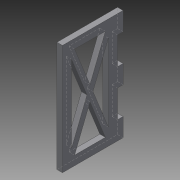
# Autodesk Inventor part: Back Plate
Saved by Autodesk Inventor 2015 (Build 190159000, 159)
## iProperties
Created: 2014-07-28
Part Number: Back Plate
Material: Generic
Document SubType Name: Modeling
Designer: karl
Density: 1 g/cm^3
Appearance: Default
Author: karl
Autodesk Inventor part; units mm, degrees
ref_plane "YZ Plane" through (0, 0, 0) normal (1, 0, 0) x (0, 1, 0)
ref_plane "XZ Plane" through (0, 0, 0) normal (0, 1, 0) x (-1, 0, 0)
ref_plane "XY Plane" through (0, 0, 0) normal (0, 0, 1) x (1, 0, 0)
sketch "Sketch1" plane through (0, 0, 0) normal (1, 0, 0) x (0, 1, 0)
  line L0 (15, 30) -> (-15, 30)
  line L1 (-15, 30) -> (-15, -30)
  line L2 (-15, -30) -> (15, -30)
  line L3 (15, -30) -> (15, 30)
  line L4 (15, 30) -> (-15, -30) construction
  line L5 (-15, 30) -> (15, -30) construction
  line L6 (15, 30) -> (18, 30)
  line L7 (18, 30) -> (18, 20)
  line L8 (18, 20) -> (15, 20)
  line L9 (15, 20) -> (15, 30)
  line L10 (15, -30) -> (18, -30)
  line L11 (18, -30) -> (18, -20)
  line L12 (18, -20) -> (15, -20)
  line L13 (15, -20) -> (15, -30)
  line L14 (15, 5) -> (18, 5)
  line L15 (18, 5) -> (18, -5)
  line L16 (18, -5) -> (15, -5)
  line L17 (15, -5) -> (15, 5)
  point P0 (0, 0)
  point P1 (18, 0)
  point P2 (0, 0)
  dimension "d0" = 30
  dimension "d1" = 60
  dimension "d2" = 3
  dimension "d3" = 10
  dimension "d4" = 3
  dimension "d5" = 10
  dimension "d6" = 3
  dimension "d7" = 10
  constraints: 36 end point, 8 parallel, 4 horizontal, 4 midpoint, 4 perpendicular, 1 horizontal alignment, 1 point on line
  measures "d0" distance of L2.end L1.end
  measures "d1" distance of L0.end L1.end
  measures "d2" distance of L7.end L8.end
  measures "d3" distance of L6.end L7.end
  measures "d4" distance of L12.end L11.end
  measures "d5" distance of L11.end L10.end
  measures "d6" distance of L15.end L16.end
  measures "d7" distance of L14.end L15.end
extrude "Extrusion1" add sketch "Sketch1" along normal blind 3
sketch "Sketch2" plane through (0, 0, 0) normal (-1, 0, 0) x (0, 0, 1)
  line L0 (25, 10) -> (-25, 10)
  line L1 (-25, 10) -> (-25, -10)
  line L2 (-25, -10) -> (25, -10)
  line L3 (25, -10) -> (25, 10)
  line L4 (25, 10) -> (-25, -10) construction
  line L5 (-25, 10) -> (25, -10) construction
  line L6 (30, -15) -> (-30, -15) projected
  line L7 (-30, -15) -> (-30, 18) projected
  point P0 (0, 0)
  dimension "d10" = 5
  dimension "d11" = 5
  constraints: 12 end point, 2 midpoint, 2 parallel, 1 horizontal, 1 perpendicular
  measures "d10" distance between parallel lines of L6 L2
  measures "d11" distance between parallel lines of L7 L1
extrude "Extrusion2" cut sketch "Sketch2" against normal blind 3
sketch "Sketch3" plane through (0, 0, 0) normal (-1, 0, 0) x (0, 0, 1)
  line L0 (-25, -10) -> (-25, 10) projected
  line L1 (-25, 10) -> (25, 10) projected
  line L2 (25, 10) -> (25, -10) projected
  line L3 (25, -10) -> (-25, -10) projected
  line L4 (-30, -15) -> (-30, 18) projected
  line L5 (30, -15) -> (-30, -15) projected
  line L6 (30, 18) -> (30, -15) projected
  line L7 (20, 18) -> (30, 18) projected
  line L8 (20, 15) -> (20, 18) projected
  line L9 (5, 15) -> (20, 15) projected
  line L10 (5, 18) -> (5, 15) projected
  line L11 (-5, 18) -> (5, 18) projected
  line L12 (-5, 15) -> (-5, 18) projected
  line L13 (-20, 15) -> (-5, 15) projected
  line L14 (-20, 18) -> (-20, 15) projected
  line L15 (-30, 18) -> (-20, 18) projected
  line L16 (25.5571, 8.6073) -> (-24.4429, -11.3927)
  line L17 (-24.4429, -11.3927) -> (-25.5571, -8.6073)
  line L18 (-25.5571, -8.6073) -> (24.4429, 11.3927)
  line L19 (24.4429, 11.3927) -> (25.5571, 8.6073)
  line L20 (25.5571, 8.6073) -> (-25.5571, -8.6073) construction
  line L21 (-24.4429, -11.3927) -> (24.4429, 11.3927) construction
  line L22 (-25.5571, 8.6073) -> (24.4429, -11.3927)
  line L23 (24.4429, -11.3927) -> (25.5571, -8.6073)
  line L24 (25.5571, -8.6073) -> (-24.4429, 11.3927)
  line L25 (-24.4429, 11.3927) -> (-25.5571, 8.6073)
  line L26 (-25.5571, 8.6073) -> (25.5571, -8.6073) construction
  line L27 (24.4429, -11.3927) -> (-24.4429, 11.3927) construction
  point P0 (0, 0)
  dimension "d14" = 3
  dimension "d15" = 3
  constraints: 24 end point, 4 midpoint, 4 parallel, 2 perpendicular
  measures "d14" distance of L16.end L17.end
  measures "d15" distance of L23.end L22.end
extrude "Extrusion3" add sketch "Sketch3" against normal blind 3 contours L17 L18 L0 | L0 L18 L22 L16 L3 | L3 L16 L17 | L22 L25 L0 | L0 L1 L24 L18 L22 | L18 L24 L16 L22 | L22 L16 L24 L2 L3 | L3 L23 L22 | L25 L24 L1 | L18 L1 L2 L16 L24 | L2 L24 L23 | L18 L19 L1 | L2 L19 L16
body "Solid1"
